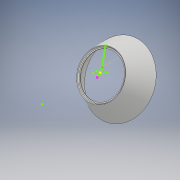
# Autodesk Inventor part: A1_V1_M2_dropArm_WOK_meso_tall_VIS_FULL
Saved by Autodesk Inventor 2018 (Build 220112000, 112)
## iProperties
Created: 2018-04-20
Part Number: A1_V1_M2_dropArm_WOK_meso_tall_VIS_FULL
Material: Generic
Document SubType Name: Modeling
Designer: McCormick Lab
Density: 1 g/cm^3
Appearance: Default
Author: McCormick Lab
Autodesk Inventor part; units mm, degrees
ref_plane "YZ Plane" through (0, 0, 0) normal (1, 0, 0) x (0, 1, 0)
ref_plane "XZ Plane" through (0, 0, 0) normal (0, 1, 0) x (-1, 0, 0)
ref_plane "XY Plane" through (0, 0, 0) normal (0, 0, 1) x (1, 0, 0)
sketch "Sketch68" plane through (0, 0, 0) normal (1, 0, 0) x (0, 1, 0)
  line L0 (1, 4.6737) -> (23, 4.6737) construction
  line L1 (7.0021, -2.9903) -> (-7.0029, -0.0135)
  line L2 (7.2385, 26.8729) -> (5.7713, 27.1847)
  line L3 (2.4565, 4.3755) -> (1, 4.6737)
  line L4 (5.7713, 27.1847) -> (1, 4.6737)
  line L5 (7.2385, 26.8729) -> (2.4565, 4.3755)
  point P0 (0, 0)
  point P1 (2.225, 5.1772)
  constraints: 12 end point, 1 horizontal
sketch "Sketch184" plane through (0, 0, 0) normal (1, 0, 0) x (0, 1, 0)
  arc A0 (-3.5, -3.0972) -> (0, -1.6204) centre (-4.281, 3.6397) ccw
  arc A1 (0, -1.6204) -> (2.2822, 2) centre (-4.3557, 3.6547) ccw
  arc A2 (2.2822, 2) -> (2.459, 4.3851) centre (-8.8285, 4.0231) ccw
  arc A3 (2.459, 4.3851) -> (2.3883, 6) centre (-72.7121, 1.9029) ccw
  line L0 (-3.5, -3.0972) -> (-3.5, -3.6807) projected
  arc A4 (2.3883, 6) -> (-3.5, -3.0972) centre (8.6947, -4.5362) ccw
  point P0 (0, 0)
  constraints: 10 point on circle, 5 centre point
sketch "Sketch213" plane through (0, 0, 0) normal (1, 0, 0) x (0, 1, 0)
  line L0 (13.3414, -11.8728) -> (-10.8201, 5)
  line L1 (46.9769, 13.1952) -> (16.4024, 18.5466)
  line L2 (-14, -25) -> (0.7357, -50.4491)
  line L3 (0.7357, -50.4491) -> (1.9473, -49.7476)
  line L4 (46.9769, 13.1952) -> (46.7355, 11.8161)
  line L5 (1.9473, -49.7476) -> (-11.7207, -26.1425)
  line L6 (-11.7207, -26.1425) -> (-10, -24)
  line L7 (-10, -24) -> (-10.853, -23.4043)
  line L8 (-10.853, -23.4043) -> (-11.992, -25.0353)
  line L9 (-11.992, -25.0353) -> (-13.0313, -25.7169)
  line L10 (-13.0313, -25.7169) -> (-11.992, -25.0353) projected
  line L11 (-13.0313, -25.7169) -> (-12.7653, -23.856)
  line L12 (-12.7653, -23.856) -> (-14, -25)
  line L13 (46.7355, 11.8161) -> (18.2275, 16.8059)
  line L14 (18.2275, 16.8059) -> (17, 15)
  line L15 (17, 15) -> (16.3637, 15.4444)
  line L16 (-11.992, -25.0353) -> (16.9748, 16.4444) projected
  line L17 (16.3637, 15.4444) -> (17.062, 16.4444)
  line L18 (17.062, 16.4444) -> (17.3561, 17.7094)
  line L19 (17.3561, 17.7094) -> (16.3637, 17.6698)
  line L20 (16.3637, 17.6698) -> (16.4024, 18.5466)
  point P0 (0, 0)
  point P1 (3.3399, -2.2736)
  point P2 (-1.2043, -8.7808)
  dimension "d600" = 1.4
  dimension "d601" = 1.4
  dimension "d603" = 1.265
  constraints: 38 end point, 1 perpendicular
  measures "d600" distance of L2.end L3.end
  measures "d601" distance of L1.start L4.end
  measures "d603" vertical distance of L18.end L17.end
revolve "Revolution5" add sketch "Sketch213" angle 360 about axis through (0, 13.3414, -11.8728) along (0, -0.8199, 0.5725) contours L4 L13 L14 L15 L17 L18 L19 L20 L1
body "Solid2"
